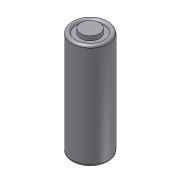
# Autodesk Inventor part: battery_A_SanyoKR1700AU
Saved by Autodesk Inventor 2014 SP1 (Build 180222100, 222)
## iProperties
Created: 2011-09-10
Part Number: battery_A_SanyoKR1700AU
Document SubType Name: Modeling
Designer: Robert Davis
Density: 3.55 g/cm^3
Material: NiCad
Mass: 36.0069 g
Surface Area: 33.0233 cm^2
Volume: 10.1428 cm^3
Appearance: Steel
Author: Robert Davis
Autodesk Inventor part; units mm, degrees
ref_plane "YZ Plane" through (0, 0, 0) normal (1, 0, 0) x (0, 1, 0)
ref_plane "XZ Plane" through (0, 0, 0) normal (0, 1, 0) x (-1, 0, 0)
ref_plane "XY Plane" through (0, 0, 0) normal (0, 0, 1) x (1, 0, 0)
sketch "Sketch1" plane through (0, 0, 0) normal (0, 0, 1) x (1, 0, 0)
  circle A0 centre (0, 0) radius 8.25
  dimension "d0" = 16.5
  constraints: 1 centre point
  measures "d0" diameter of A0
extrude "cylinder" add sketch "Sketch1" along normal mid plane 48.5
sketch "Sketch7" plane through (0, 0, 24.25) normal (0, 0, 1) x (1, 0, 0)
  circle A0 centre (0, 0) radius 8.25 projected
  circle A1 centre (0, 0) radius 4.25
  circle A2 centre (0, 0) radius 8.25
  dimension "d17" = 8.5
  constraints: 2 centre point
  measures "d17" diameter of A1
extrude "button" cut sketch "Sketch7" against normal blind 2
fillet "Fillet1" radius 1 1 edges at (-8.25, 0, -24.25)
sketch "Sketch8" plane through (0, 0, 0) normal (0, 1, 0) x (-1, 0, 0)
  arc A0 (-6.25, 22.25) -> (-8.25, 22.25) centre (-7.25, 22.25) ccw
  line L0 (-8.25, 22.25) -> (8.25, 22.25) projected
  line L1 (-6.25, 23.25) -> (-8.25, 23.25)
  line L2 (0, -34.65) -> (0, 34.65) projected
  point P0 (0, 0)
  dimension "d20" = 1
  dimension "d21" = 8.25
  constraints: 3 point on line, 2 end point, 2 point on circle, 1 centre point
  measures "d20" radius of A0
  measures "d21" horizontal distance of point (0, 0) A0.end
revolve "rolled_edge" add sketch "Sketch8" angle 360 about axis through (0, 0, 0) along (0, 0, 1)
body "Solid1"
